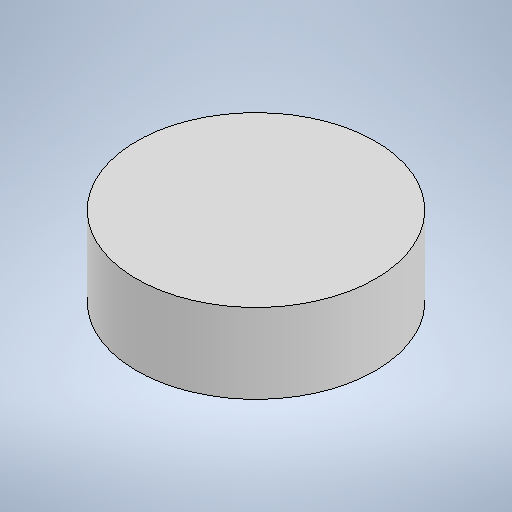
# Autodesk Inventor part: PRS 940-81-01 DIM Filter column D1200
Saved by Autodesk Inventor 2025.1 (Build 291241020, 241B)
## iProperties
Created: 2025-02-12
Part Number: PRS 940-81-01 DIM Filter column D1200
Material: Generic
Document SubType Name: Modeling
Designer: pokla
Density: 1 g/cm^3
Appearance: Default
Mass: 2.47582e+06 g
Surface Area: 99298.1 cm^2
Volume: 2.47582e+06 cm^3
MAIN_filter_diam: 1200,000 mm
MAIN_hight: 2310.000 mm
Accsess_hatch_diameter: 530,000 mm
Accsess_hatch_lenght: 120,000 mm
Charging_hatch_width: 400,000 mm
Charging_hatch_hight: 180,000 mm
Charging_hatch_lenght: 120,000 mm
Author: pokla
Autodesk Inventor part; units mm, degrees
ref_plane "YZ Plane" through (0, 0, 0) normal (1, 0, 0) x (0, 1, 0)
ref_plane "XZ Plane" through (0, 0, 0) normal (0, 1, 0) x (-1, 0, 0)
ref_plane "XY Plane" through (0, 0, 0) normal (0, 0, 1) x (1, 0, 0)
sketch "Sketch1" plane through (0, 0, 0) normal (0, 0, 1) x (1, 0, 0)
  circle A0 centre (0, 0) radius 44.45
  circle A1 centre (0, 0) radius 41.45
  circle A2 centre (0, 0) radius 600
  circle A3 centre (144.9387, 540.9185) radius 100
  circle A4 centre (-144.9387, 540.9185) radius 100
  circle A5 centre (-395.9798, 395.9798) radius 100
  circle A6 centre (-540.9185, 144.9387) radius 100
  circle A7 centre (-540.9185, -144.9387) radius 100
  circle A8 centre (-395.9798, -395.9798) radius 100
  circle A9 centre (-144.9387, -540.9185) radius 100
  circle A10 centre (144.9387, -540.9185) radius 100
  circle A11 centre (395.9798, -395.9798) radius 100
  circle A12 centre (540.9185, -144.9387) radius 100
  circle A13 centre (230, 398.3717) radius 100
  circle A14 centre (0, 460) radius 100
  circle A15 centre (-230, 398.3717) radius 100
  circle A16 centre (-398.3717, 230) radius 100
  circle A17 centre (-460, 0) radius 100
  circle A18 centre (-398.3717, -230) radius 100
  circle A19 centre (-230, -398.3717) radius 100
  circle A20 centre (0, -460) radius 100
  circle A21 centre (230, -398.3717) radius 100
  circle A22 centre (398.3717, -230) radius 100
  circle A23 centre (-212.132, 212.132) radius 100
  circle A24 centre (-289.7777, 77.6457) radius 100
  circle A25 centre (-289.7777, -77.6457) radius 100
  circle A26 centre (-212.132, -212.132) radius 100
  circle A27 centre (-77.6457, -289.7777) radius 100
  circle A28 centre (77.6457, -289.7777) radius 100
  circle A29 centre (212.132, -212.132) radius 100
  circle A30 centre (289.7777, -77.6457) radius 100
  circle A31 centre (98.9949, 98.9949) radius 100
  circle A32 centre (289.7777, 77.6457) radius 100
  circle A33 centre (212.132, 212.132) radius 100
  circle A34 centre (-98.9949, 98.9949) radius 100
  circle A35 centre (-98.9949, -98.9949) radius 100
  circle A36 centre (98.9949, -98.9949) radius 100
  circle A37 centre (460, 0) radius 100
  circle A38 centre (398.3717, 230) radius 100
  circle A39 centre (77.6457, 289.7777) radius 100
  circle A40 centre (-77.6457, 289.7777) radius 100
  circle A41 centre (540.9185, 144.9387) radius 100
  circle A42 centre (395.9798, 395.9798) radius 100
  line L0 (0, 0) -> (-600, 0) construction
  line L1 (0, 0) -> (-540.9185, 144.9387) construction
  line L2 (-460, 0) -> (0, 0) construction
  line L3 (0, 0) -> (-289.7777, -77.6457) construction
  line L4 (-98.9949, -98.9949) -> (0, 0) construction
  dimension "d2" = 1200
  dimension "d0" = 88.9
  dimension "d1" = 3
  dimension "d5" = 360
  dimension "d9" = 360
  dimension "d11" = 200
  dimension "d14" = 360
  dimension "d18" = 360
  dimension "d20" = 15
  dimension "d21" = 0
  dimension "d22" = 15
  dimension "d23" = 45
  dimension "d24" = 140
  dimension "d25" = 300
  dimension "d26" = 460
  dimension "d27" = 560
  constraints: 42 centre point, 10 end point, 3 equal radius, 2 coincident, 1 horizontal, 1 horizontal alignment, 86 other
  measures "d0" diameter of A0
  measures "d1" radial gap between concentric circles of A0 A1
  measures "d11" diameter of A13
  measures "d20" angle of L0 L1
  measures "d21" distance between parallel lines of L0 L2
  measures "d22" angle of L3 L2
  measures "d23" angle of L4 L2
  measures "d24" distance of L4.start L0.start
  measures "d25" distance of L0.start L3.end
  measures "d26" distance of L2.start L0.start
  measures "d27" distance of L0.start L1.end
sketch "Sketch2" plane through (0, 0, 0) normal (0, 0, 1) x (1, 0, 0)
  point P0 (0, 0)
  point P1 (-98.9949, -98.9949)
  point P2 (98.9949, -98.9949)
  point P3 (98.9949, 98.9949)
  point P4 (-98.9949, 98.9949)
  point P5 (-77.6457, 289.7777)
  point P6 (77.6457, 289.7777)
  point P7 (212.132, 212.132)
  point P8 (289.7777, 77.6457)
  point P9 (289.7777, -77.6457)
  point P10 (212.132, -212.132)
  point P11 (77.6457, -289.7777)
  point P12 (-77.6457, -289.7777)
  point P13 (0, -460)
  point P14 (230, -398.3717)
  point P15 (144.9387, -540.9185)
  point P16 (395.9798, -395.9798)
  point P17 (398.3717, -230)
  point P18 (540.9185, -144.9387)
  point P19 (460, 0)
  point P20 (540.9185, 144.9387)
  point P21 (398.3717, 230)
  point P22 (395.9798, 395.9798)
  point P23 (230, 398.3717)
  point P24 (144.9387, 540.9185)
  point P25 (0, 460)
  point P26 (-144.9387, 540.9185)
  point P27 (-230, 398.3717)
  point P28 (-212.132, 212.132)
  point P29 (-289.7777, 77.6457)
  point P30 (-289.7777, -77.6457)
  point P31 (-212.132, -212.132)
  point P32 (-398.3717, 230)
  point P33 (-395.9798, 395.9798)
  point P34 (-540.9185, 144.9387)
  point P35 (-460, 0)
  point P36 (-540.9185, -144.9387)
  point P37 (-398.3717, -230)
  point P38 (-395.9798, -395.9798)
  point P39 (-230, -398.3717)
  point P40 (-144.9387, -540.9185)
sketch "Sketch3" plane through (0, 0, 0) normal (0, 0, 1) x (1, 0, 0)
  circle A0 centre (0, 0) radius 15
  dimension "d28" = 30
  constraints: 1 centre point, 1 coincident
  measures "d28" diameter of A0
extrude "Extrusion1" add sketch "Sketch3" along normal blind 10
sketch "Sketch4" plane through (0, 0, 0) normal (1, 0, 0) x (0, 1, 0)
  line L0 (606, 2056.7108) -> (600, 2056.7108)
  line L1 (600, 2056.7108) -> (600, 253.2892)
  line L2 (600, 253.2892) -> (606, 253.2892)
  line L3 (606, 253.2892) -> (606, 2056.7108)
  line L4 (0, 253.2892) -> (0, 1462.6576)
  line L5 (606, 253.2892) -> (606, 223.2892)
  arc A0 (552, 134.4973) -> (606, 223.2892) centre (506, 223.2892) ccw
  arc A1 (0, 0) -> (552, 134.4973) centre (0, 1200) ccw
  line L6 (0, 898.5253) -> (0, -391.9469)
  arc A2 (0, 6) -> (549.24, 139.8248) centre (0, 1200) ccw
  arc A3 (549.24, 139.8248) -> (600, 223.2892) centre (506, 223.2892) ccw
  line L7 (600, 223.2892) -> (600, 253.2892)
  line L8 (600, 253.2892) -> (606, 253.2892)
  line L9 (0, 6) -> (0, 0)
  line L10 (600, 2056.7108) -> (600, 2086.7108)
  arc A4 (600, 2086.7108) -> (549.24, 2170.1752) centre (506, 2086.7108) ccw
  arc A5 (549.24, 2170.1752) -> (0, 2304) centre (0, 1110) ccw
  line L11 (0, 2304) -> (0, 2310)
  arc A6 (552, 2175.5027) -> (0, 2310) centre (0, 1110) ccw
  arc A7 (606, 2086.7108) -> (552, 2175.5027) centre (506, 2086.7108) ccw
  line L12 (606, 2086.7108) -> (606, 2056.7108)
  line L13 (0, 2304) -> (0, 6)
  point P0 (0, 0)
  point P1 (600, 253.2892)
  point P2 (603, 253.2892)
  point P3 (0, 253.2892)
  point P4 (0, 253.2892)
  point P5 (0, 3)
  point P6 (0, 0)
  dimension "d31" = 6
  dimension "d32" = 1803.4216
  dimension "d33" = 1200
  dimension "d37" = 100
  dimension "d38" = 30
  dimension "d39" = 1200
  dimension "d40" = 6
  dimension "d41" = 1200
  dimension "d42" = 253.2892
  constraints: 28 end point, 16 point on circle, 8 centre point, 6 tangent, 5 vertical, 4 equal radius, 3 coincident, 3 equal length, 3 midpoint, 3 parallel, 2 collinear, 2 horizontal, 2 horizontal alignment, 1 line through centre, 1 perpendicular, 1 point on line, 1 vertical alignment, 2 other
  measures "d31" distance between parallel lines of L1 L3
  measures "d32" distance of L2.end L0.start
  measures "d33" diameter of L1 L4
  measures "d37" radius of A0
  measures "d38" distance of L5.start L5.end
  measures "d39" radius of A1
  measures "d40" radial gap between concentric circles of A1 A2
  measures "d41" diameter of L7 L6
  measures "d42" distance of L9.end point (0, 253.289)
revolve "Revolution1" [suppressed]
equation "\"d32\" = d35 - 2 * d36"
equation "\"d33\" = d34"
equation "\"d39\" = d41"
equation "\"MAIN_filter_diam\" = 1200"
equation "\"MAIN_hight\" = 2310"
equation "\"Accsess_hatch_lenght\" = 120"
equation "\"Accsess_hatch_diameter\" = 530"
equation "\"Charging_hatch_width\" = 400"
equation "\"Charging_hatch_hight\" = 180"
equation "\"Charging_hatch_lenght\" = 120"
equation "\"d35\" = 2310"
equation "\"d36\" = 253.289193"
equation "\"d34\" = 1200"
body "Solid1"
